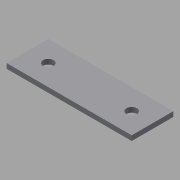
# Autodesk Inventor part: Small Arm
Saved by Autodesk Inventor 2013 (Build 170138000, 138)
## iProperties
Created: 2013-02-08
Part Number: Small Arm
Material: Generic
Document SubType Name: Modeling
Designer: Naphat
Density: 1 g/cm^3
Author: Naphat
Autodesk Inventor part; units mm, degrees
ref_plane "YZ Plane" through (0, 0, 0) normal (1, 0, 0) x (0, 1, 0)
ref_plane "XZ Plane" through (0, 0, 0) normal (0, 1, 0) x (-1, 0, 0)
ref_plane "XY Plane" through (0, 0, 0) normal (0, 0, 1) x (1, 0, 0)
sketch "Sketch1" plane through (0, 0, 0) normal (0, 1, 0) x (-1, 0, 0)
  line L0 (0, 0) -> (0, 25.4)
  line L1 (0, 25.4) -> (76.2, 25.4)
  line L2 (76.2, 25.4) -> (76.2, 0)
  line L3 (76.2, 0) -> (0, 0)
  dimension "d0" = 25.4
  dimension "d1" = 76.2
  constraints: 8 end point, 2 perpendicular, 1 parallel, 1 vertical
  measures "d0" distance of L0.start L0.end
  measures "d1" distance of L0.end L1.end
extrude "Extrusion1" add sketch "Sketch1" along normal blind 3
sketch "Sketch2" plane through (0, 3, 0) normal (0, 1, 0) x (1, 0, 0)
  line L0 (0, 0) -> (-76.2, 0) projected
  line L1 (-76.2, -25.4) -> (0, -25.4) projected
  line L2 (-76.2, -12.7) -> (0, -12.7) construction
  line L3 (-76.2, -25.4) -> (-63.5, -25.4) construction
  line L4 (-63.5, -25.4) -> (-63.5, 0) construction
  line L5 (0, 0) -> (-12.7, 0) construction
  line L6 (-12.7, 0) -> (-12.7, -25.4) construction
  circle A0 centre (-63.5, -12.7) radius 3.175
  circle A1 centre (-12.7, -12.7) radius 3.175
  line L7 (-76.2, 0) -> (-76.2, -12.7) construction
  line L8 (0, -12.7) -> (0, 0) construction
  line L9 (0, -25.4) -> (0, 0) projected
  line L10 (-76.2, 0) -> (-76.2, -25.4) projected
  dimension "d5" = 12.7
  dimension "d7" = 12.7
  dimension "d8" = 6.35
  dimension "d9" = 6.35
  dimension "d10" = 12.7
  dimension "d11" = 12.7
  constraints: 14 end point, 4 point on line, 3 perpendicular, 2 centre point, 2 midpoint
  measures "d5" distance of L1.start L3.end
  measures "d7" distance of L0.start L5.end
  measures "d8" diameter of A0
  measures "d9" diameter of A1
  measures "d10" distance of L0.end L2.start
  measures "d11" distance of L2.end L0.start
hole "Hole1" at (-63.5, 3, 12.7) at (-12.7, 3, 12.7) direction (0, -1, 0) diameter 6.35 depth 25.4 tip angle 118
equation "\"d5\" = d7"
equation "\"d8\" = d9"
body "Solid1"
